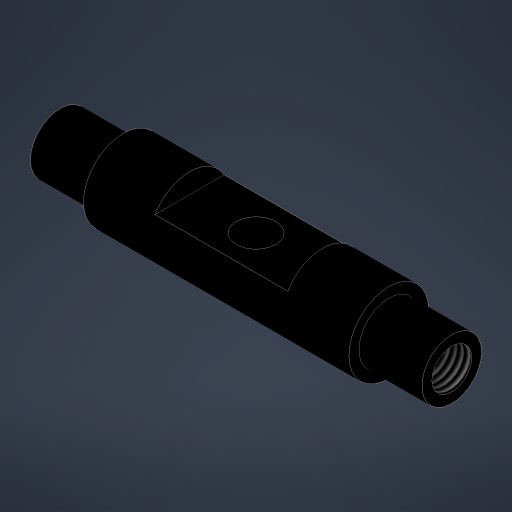
# Autodesk Inventor part: Z25_Spacer
Saved by Autodesk Inventor 2025 (Build 290162010, 162A)
## iProperties
Created: 2023-02-13
Part Number: Z25_Spacer
Material: Aluminum 6061
Document SubType Name: Modeling
Designer: dzw04
Density: 2.7 g/cm^3
Appearance: Anodized - Black
Author: dzw04
Autodesk Inventor part; units mm, degrees
ref_plane "YZ Plane" through (0, 0, 0) normal (1, 0, 0) x (0, 1, 0)
ref_plane "XZ Plane" through (0, 0, 0) normal (0, 1, 0) x (-1, 0, 0)
ref_plane "XY Plane" through (0, 0, 0) normal (0, 0, 1) x (1, 0, 0)
sketch "Sketch1" plane through (0, 0, 0) normal (1, 0, 0) x (0, 1, 0)
  circle A0 centre (0, 0) radius 3
  dimension "d0" = 6
  constraints: 1 centre point, 1 coincident
  measures "d0" diameter of A0
extrude "Extrusion1" add sketch "Sketch1" along normal mid plane 29.5
sketch "Sketch2" plane through (14.75, 0, 0) normal (1, 0, 0) x (0, 0, -1)
  circle A0 centre (0, 0) radius 2.25
  circle A1 centre (0, 0) radius 1.5
  circle A2 centre (0, 0) radius 3
  dimension "d3" = 4.5
  dimension "d4" = 3
  constraints: 3 centre point, 3 coincident
  measures "d3" diameter of A0
  measures "d4" diameter of A1
extrude "Extrusion2" cut sketch "Sketch2" against normal blind 4.75
sketch "Sketch3" plane through (-14.75, 0, 0) normal (-1, 0, 0) x (0, 0, 1)
  circle A0 centre (0, 0) radius 2.25
  circle A1 centre (0, 0) radius 1.5
  circle A2 centre (0, 0) radius 3
  dimension "d7" = 4.5
  dimension "d8" = 3
  dimension "d9" = 6
  constraints: 3 centre point, 3 coincident
  measures "d7" diameter of A0
  measures "d8" diameter of A1
  measures "d9" diameter of A2
extrude "Extrusion3" cut sketch "Sketch3" against normal blind 4.75
sketch "Sketch4" plane through (0, 0, 0) normal (1, 0, 0) x (0, 1, 0)
  circle A0 centre (0, 0) radius 3 projected
  line L0 (3, 0) -> (1.5, 0)
  line L1 (1.5, 3.5) -> (3, 3.5)
  line L2 (3, 3.5) -> (3, -3.5)
  line L3 (3, -3.5) -> (1.5, -3.5)
  line L4 (1.5, -3.5) -> (1.5, 3.5)
  circle A1 centre (0, 0) radius 2.25 projected
  line L5 (1.5, 3.5) -> (3, -3.5) construction
  line L6 (3, 3.5) -> (1.5, -3.5) construction
  point P0 (2.25, 0)
  dimension "d12" = 1.5
  dimension "d13" = 7
  constraints: 14 end point, 3 midpoint, 2 horizontal, 2 horizontal alignment, 2 parallel, 1 perpendicular, 2 other
  measures "d12" distance of L0.start L0.end
  measures "d13" distance of L1.end L2.end
extrude "Extrusion4" cut sketch "Sketch4" along normal mid plane 10 contours L0 A1 L4 A0 | L2 L3 L4 A0 | A0 L4 A1 L0 | A0 L4 L1 L2 | A1 L4 L0 | L0 L4 A1
sketch "Sketch5" plane through (-5, 1.5, -2.5981) normal (0, 1, 0) x (1, 0, 0)
  circle A0 centre (5, -2.5981) radius 1.5
  dimension "d16" = 3
  constraints: 1 centre point, 1 coincident
  measures "d16" diameter of A0
extrude "Extrusion5" cut sketch "Sketch5" against normal through all
thread "Thread1" size "M3x0.5" class "6H" standard "ANSI Metric M Profile" full length
thread "Thread2" size "M3x0.5" class "6H" standard "ANSI Metric M Profile" full length
sketch "Sketch6" plane through (10, 0, 0) normal (1, 0, 0) x (0, 0, -1)
  circle A0 centre (0, 0) radius 1.5
  constraints: 1 centre point, 1 coincident
extrude "Extrusion6" cut sketch "Sketch6" against normal blind 2
sketch "Sketch7" plane through (-10, 0, 0) normal (-1, 0, 0) x (0, 0, 1)
  circle A0 centre (0, 0) radius 1.5
  constraints: 1 centre point, 1 coincident
extrude "Extrusion7" cut sketch "Sketch7" against normal blind 2
body "Solid1"
